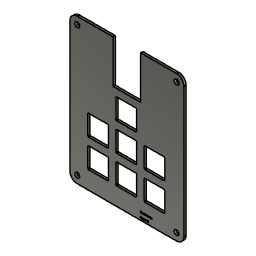
zohair plate v1 (Autodesk Fusion 360 design; units mm, degrees)
Autodesk Fusion 360 part; units mm, degrees
sketch "plate-2025-02-18T21_41_00.606Z" plane through (0, 0, 0) normal (0, 1, 0) x (1, 0, 0)
  line L0 (86.175, -124.775) -> (73.175, -124.775)
  line L1 (86.175, -110.775) -> (73.175, -110.775)
  line L2 (86.675, -124.275) -> (86.675, -111.275)
  line L3 (72.675, -124.275) -> (72.675, -111.275)
  arc A0 (86.175, -124.775) -> (86.675, -124.275) centre (86.175, -124.275) ccw
  arc A1 (72.675, -124.275) -> (73.175, -124.775) centre (73.175, -124.275) ccw
  arc A2 (86.675, -111.275) -> (86.175, -110.775) centre (86.175, -111.275) ccw
  arc A3 (73.175, -110.775) -> (72.675, -111.275) centre (73.175, -111.275) ccw
  line L4 (105.225, -105.725) -> (92.225, -105.725)
  line L5 (105.225, -91.725) -> (92.225, -91.725)
  line L6 (105.725, -105.225) -> (105.725, -92.225)
  line L7 (91.725, -105.225) -> (91.725, -92.225)
  arc A4 (105.225, -105.725) -> (105.725, -105.225) centre (105.225, -105.225) ccw
  arc A5 (91.725, -105.225) -> (92.225, -105.725) centre (92.225, -105.225) ccw
  arc A6 (105.725, -92.225) -> (105.225, -91.725) centre (105.225, -92.225) ccw
  arc A7 (92.225, -91.725) -> (91.725, -92.225) centre (92.225, -92.225) ccw
  line L8 (86.175, -105.725) -> (73.175, -105.725)
  line L9 (86.175, -91.725) -> (73.175, -91.725)
  line L10 (86.675, -105.225) -> (86.675, -92.225)
  line L11 (72.675, -105.225) -> (72.675, -92.225)
  arc A8 (86.175, -105.725) -> (86.675, -105.225) centre (86.175, -105.225) ccw
  arc A9 (72.675, -105.225) -> (73.175, -105.725) centre (73.175, -105.225) ccw
  arc A10 (86.675, -92.225) -> (86.175, -91.725) centre (86.175, -92.225) ccw
  arc A11 (73.175, -91.725) -> (72.675, -92.225) centre (73.175, -92.225) ccw
  line L12 (67.125, -105.725) -> (54.125, -105.725)
  line L13 (67.125, -91.725) -> (54.125, -91.725)
  line L14 (67.625, -105.225) -> (67.625, -92.225)
  line L15 (53.625, -105.225) -> (53.625, -92.225)
  arc A12 (67.125, -105.725) -> (67.625, -105.225) centre (67.125, -105.225) ccw
  arc A13 (53.625, -105.225) -> (54.125, -105.725) centre (54.125, -105.225) ccw
  arc A14 (67.625, -92.225) -> (67.125, -91.725) centre (67.125, -92.225) ccw
  arc A15 (54.125, -91.725) -> (53.625, -92.225) centre (54.125, -92.225) ccw
  line L16 (105.225, -86.675) -> (92.225, -86.675)
  line L17 (105.225, -72.675) -> (92.225, -72.675)
  line L18 (105.725, -86.175) -> (105.725, -73.175)
  line L19 (91.725, -86.175) -> (91.725, -73.175)
  arc A16 (105.225, -86.675) -> (105.725, -86.175) centre (105.225, -86.175) ccw
  arc A17 (91.725, -86.175) -> (92.225, -86.675) centre (92.225, -86.175) ccw
  arc A18 (105.725, -73.175) -> (105.225, -72.675) centre (105.225, -73.175) ccw
  arc A19 (92.225, -72.675) -> (91.725, -73.175) centre (92.225, -73.175) ccw
  line L20 (86.175, -86.675) -> (73.175, -86.675)
  line L21 (86.175, -72.675) -> (73.175, -72.675)
  line L22 (86.675, -86.175) -> (86.675, -73.175)
  line L23 (72.675, -86.175) -> (72.675, -73.175)
  arc A20 (86.175, -86.675) -> (86.675, -86.175) centre (86.175, -86.175) ccw
  arc A21 (72.675, -86.175) -> (73.175, -86.675) centre (73.175, -86.175) ccw
  arc A22 (86.675, -73.175) -> (86.175, -72.675) centre (86.175, -73.175) ccw
  arc A23 (73.175, -72.675) -> (72.675, -73.175) centre (73.175, -73.175) ccw
  line L24 (67.125, -86.675) -> (54.125, -86.675)
  line L25 (67.125, -72.675) -> (54.125, -72.675)
  line L26 (67.625, -86.175) -> (67.625, -73.175)
  line L27 (53.625, -86.175) -> (53.625, -73.175)
  arc A24 (67.125, -86.675) -> (67.625, -86.175) centre (67.125, -86.175) ccw
  arc A25 (53.625, -86.175) -> (54.125, -86.675) centre (54.125, -86.175) ccw
  arc A26 (67.625, -73.175) -> (67.125, -72.675) centre (67.125, -73.175) ccw
  arc A27 (54.125, -72.675) -> (53.625, -73.175) centre (54.125, -73.175) ccw
  line L28 (41.585, -158.66) -> (118.61, -158.66)
  line L29 (118.61, -158.66) -> (118.61, -60.635)
  line L30 (118.61, -60.635) -> (41.585, -60.635)
  line L31 (41.585, -60.635) -> (41.585, -158.66)
  line L32 (70.845, -158.66) -> (89.345, -158.66)
  line L33 (89.345, -158.66) -> (89.345, -127.66)
  line L34 (89.345, -127.66) -> (70.845, -127.66)
  line L35 (70.845, -127.66) -> (70.845, -158.66)
  circle A28 centre (46.585, -153.66) radius 1.7
  circle A29 centre (113.61, -153.66) radius 1.7
  circle A30 centre (46.585, -65.635) radius 1.7
  circle A31 centre (113.61, -65.635) radius 1.7
  dimension "d1" = 77.025
  dimension "d2" = 98.025
  dimension "d3" = 12.04
  dimension "d4" = 12.04
  dimension "d7" = 18.5
  dimension "d8" = 31
  dimension "d9" = 29.26
  dimension "d10" = 3.4
  dimension "d11" = 5
  dimension "d12" = 5
  dimension "d13" = 3.4
  dimension "d14" = 5
  dimension "d15" = 5
  dimension "d16" = 3.4
  dimension "d17" = 5
  dimension "d18" = 5
  dimension "d19" = 3.4
  dimension "d20" = 5
  dimension "d21" = 5
  constraint horizontal L28
  constraint vertical L29
  constraint horizontal L30
  constraint vertical L31
  constraint horizontal L32
  constraint vertical L33
  constraint horizontal L34
  constraint vertical L35
  constraint coincident L28 L32.start
  measures "d1" distance of L28.start L28.end
  measures "d2" distance of L28.start L30.end
  measures "d3" distance of L27 L31
  measures "d4" distance of L25 L30
  measures "d7" distance of L32.start L32.end
  measures "d8" distance of L32.start L34.end
  measures "d9" distance of L31 L35
  measures "d10" diameter of A28
  measures "d11" distance of L28 A28.centre
  measures "d12" distance of L31 A28.centre
  measures "d13" diameter of A29
  measures "d14" distance of L29 A29.centre
  measures "d15" distance of L28 A29.centre
  measures "d16" diameter of A30
  measures "d17" distance of L31 A30.centre
  measures "d18" distance of L30 A30.centre
  measures "d19" diameter of A31
  measures "d20" distance of L30 A31.centre
  measures "d21" distance of L29 A31.centre
extrude "Extrude1" add sketch "plate-2025-02-18T21_41_00.606Z" along normal blind 1.5 contours L28 L29 L30 L31 L33 L34 L35
sketch "Sketch2" plane through (0, 0, 0) normal (0, 1, 0) x (1, 0, 0)
sketch "Sketch3" plane through (0, 0, 0) normal (0, 1, 0) x (1, 0, 0)
extrude "Extrude2" add 1 faces at (83.1783, 1, 127.66) along direction (0, 0, 1) blind 5
extrude "Extrude3" cut 1 faces at (83.1783, 1, 132.66) along direction (0, 0, -1) blind 3
fillet "Fillet1" radius 5 4 edges at (118.61, 0.75, 60.635) (41.585, 0.75, 60.635) (41.585, 0.75, 158.66) (118.61, 0.75, 158.66)
sketch "Sketch4" plane through (0, 0, 0) normal (0, 1, 0) x (1, 0, 0)
  line L0 (89, -61.5421) -> (100.6029, -61.5421) construction
  line L1 (100.6029, -61.5421) -> (100.6029, -66) construction
  line L2 (100.6029, -66) -> (89, -66) construction
  line L3 (89, -66) -> (89, -61.5421) construction
  dimension "d30" = 1
  text T0 "Zohair / Asim\n\nSigam 42" font "Arial" height 1 align left top in box 11.6029 x 4.4579 at (89, -61.5421) x (1, 0) y (0, -1) spacing 1 kerned
extrude "Extrude4" cut sketch "Sketch4" along normal blind 0.2 text T0
